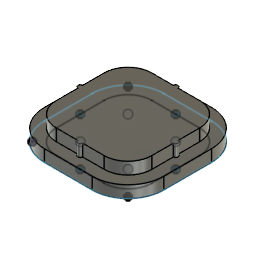
Sensor Casing Lid (Autodesk Fusion 360 design; units mm, degrees)
Autodesk Fusion 360 part; units mm, degrees
note: some values were not read from the file. Set by a fixed rule: which sketch regions a step uses.
sketch "Sketch1" plane through (0, 0, 0) normal (0, 0, 1) x (1, 0, 0)
  line L0 (10, 0) -> (30, 0)
  line L1 (40, 10) -> (40, 30)
  line L2 (30, 40) -> (10, 40)
  line L3 (0, 30) -> (0, 10)
  line L4 (10, -5) -> (30, -5)
  line L5 (45, 10) -> (45, 30)
  line L6 (30, 45) -> (10, 45)
  line L7 (-5, 30) -> (-5, 10)
  arc A0 (10, 40) -> (0, 30) centre (10, 30) ccw
  arc A1 (40, 30) -> (30, 40) centre (30, 30) ccw
  arc A2 (30, 0) -> (40, 10) centre (30, 10) ccw
  arc A3 (0, 10) -> (10, 0) centre (10, 10) ccw
  arc A4 (45, 30) -> (30, 45) centre (30, 30) ccw
  arc A5 (30, -5) -> (45, 10) centre (30, 10) ccw
  arc A6 (-5, 10) -> (10, -5) centre (10, 10) ccw
  arc A7 (10, 45) -> (-5, 30) centre (10, 30) ccw
  circle A8 centre (20, 0) radius 1
  circle A9 centre (40, 20) radius 1
  circle A10 centre (20, 40) radius 1
  circle A11 centre (0, 20) radius 1
  point P0 (40, 0)
  point P1 (0, 40)
  dimension "d1" = 40
  dimension "d2" = 40
  dimension "d3" = 10
  dimension "d4" = 15
  constraint horizontal L0
  constraint vertical L1
  constraint horizontal L2
  constraint vertical L3
  constraint horizontal L4
  constraint vertical L5
  constraint horizontal L6
  constraint vertical L7
  constraint coincident P1 L2
  constraint coincident P1 L3
  constraint tangent L2 A0
  constraint tangent L3 A0
  constraint tangent L1 A1
  constraint tangent L2 A1
  constraint equal A0 A1
  constraint coincident P0 L0
  constraint coincident P0 L1
  constraint tangent L0 A2
  constraint tangent L1 A2
  constraint equal A0 A2
  constraint coincident origin L0
  constraint coincident origin L3
  constraint tangent L0 A3
  constraint tangent L3 A3
  constraint equal A0 A3
  constraint tangent L5 A4
  constraint tangent L6 A4
  constraint tangent L4 A5
  constraint tangent L5 A5
  constraint equal A4 A5
  constraint tangent L4 A6
  constraint tangent L7 A6
  constraint equal A4 A6
  constraint tangent L6 A7
  constraint tangent L7 A7
  constraint equal A4 A7
  constraint midpoint L0 A8.centre
  constraint midpoint L1 A9.centre
  constraint midpoint L2 A10.centre
  constraint midpoint L3 A11.centre
  measures "d1" distance of origin P0
  measures "d2" distance of origin P1
  measures "d3" radius of A0
  measures "d4" radius of A4
extrude "Extrude1" add sketch "Sketch1" along normal blind 10 contours L0 L1 L2 L3 A0 A1 A2 A3 A8 A9 A10 A11 | L0 A8 | L0 A8 | L1 A9 | L1 A9 | L3 A11 | L3 A11 | L2 A10 | L2 A10
extrude "Extrude2" add sketch "Sketch1" along normal blind 5 contours L0 A8 | L1 A9 | L3 A11 | L2 A10 | L4 L5 L6 L7 A4 A5 A6 A7 picked at (19.774, -0.5035) picked at (40.3032, 20.1385) picked at (-0.4549, 20.2371) picked at (20.2754, 40.3843)
